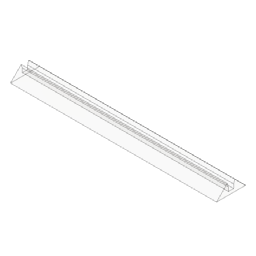
base_plexi_ledcube v2 (Autodesk Fusion 360 design; units mm, degrees)
Autodesk Fusion 360 part; units mm, degrees
sketch "Esquisse1" plane through (0, 0, 0) normal (1, 0, 0) x (0, 1, 0)
  line L0 (0, 0) -> (9.15, 0)
  line L1 (9.15, 0) -> (1.65, 7.5)
  line L2 (1.65, 7.5) -> (1.65, 2)
  line L3 (1.65, 2) -> (0, 2)
  line L4 (0, 2.5) -> (0, 20)
  line L5 (-1.65, 2) -> (0, 2)
  line L6 (0, 0) -> (-9.15, 0)
  line L7 (-1.65, 7.5) -> (-1.65, 2)
  line L8 (-9.15, 0) -> (-1.65, 7.5)
  dimension "d2" = 45
  dimension "d3" = 5.5
  dimension "d5" = 2
  dimension "d6" = 3.3
  constraint coincident L0.start L6.start
  constraint horizontal L0
  constraint vertical L2
  constraint perpendicular L2 L3
  constraint symmetric L0.start L4 L6.start
  constraint symmetric L0.end L4 L6.end
  constraint symmetric L1.end L4 L7.start
  constraint symmetric L2.end L4 L5.start
  constraint symmetric L3.end L4 L5.end
  measures "d2" angle of L0 L1
  measures "d3" distance of L1.end L2.end
  measures "d5" distance of L0 L3
  measures "d6" distance of L2 L7
extrude "Extrusion1" add sketch "Esquisse1" along normal blind 130
chamfer "Chanfrein1" distance 3 distance2 1 1 edges at (65, -1.65, 7.5) measured on face at (43.3333, -1.65, 5.6667)
chamfer "Chanfrein2" distance 1 distance2 3 1 edges at (65, 1.65, 7.5) measured on face at (43.3333, 6.65, 2.5)
component "Component" placed x (1, 0, 0) y (0, 1, 0) z (0, 0, 1) at (0, 0, 0)
